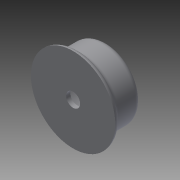
# Autodesk Inventor part: powerButtonPart2
Saved by Autodesk Inventor 2014 SP2 (Build 180246200, 246)
## iProperties
Created: 2020-04-12
Part Number: powerButtonPart2
Material: Generic
Document SubType Name: Sheet Metal
Designer: GauchoHP
Density: 1 g/cm^3
Sheet Metal Rule: Default_mm
Appearance: Default
Author: GauchoHP
Autodesk Inventor part; units mm, degrees
ref_plane "YZ Plane" through (0, 0, 0) normal (1, 0, 0) x (0, 1, 0)
ref_plane "XZ Plane" through (0, 0, 0) normal (0, 1, 0) x (-1, 0, 0)
ref_plane "XY Plane" through (0, 0, 0) normal (0, 0, 1) x (1, 0, 0)
sketch "Sketch1" plane through (0, 0, 0) normal (0, 1, 0) x (-1, 0, 0)
  circle A0 centre (0, 0) radius 9.25
  circle A1 centre (0, 0) radius 12.25
  dimension "d0" = 18.5
  dimension "d1" = 24.5
  constraints: 2 centre point, 2 coincident
  measures "d0" diameter of A0
  measures "d1" diameter of A1
extrude "Extrusion1" add sketch "Sketch1" along normal blind 10
fillet "Fillet1" radius 2 1 edges at (12.25, 10, 0)
sketch "Sketch2" plane through (0, 0, 0) normal (0, -1, 0) x (1, 0, 0)
  circle A0 centre (0, 0) radius 9.25 projected
  circle A1 centre (0, 0) radius 12.25 projected
  circle A2 centre (0, 0) radius 15
  circle A3 centre (0, 0) radius 2.5
  dimension "d6" = 30
  dimension "d9" = 5
  constraints: 2 centre point, 2 coincident
  measures "d6" diameter of A2
  measures "d9" diameter of A3
extrude "Extrusion2" add sketch "Sketch2" along normal blind 2 contours A0 | A1 | A2
fillet "Fillet3" radius 2 2 edges at (-15, 0, 0) (12.25, 0, 0)
sketch "Sketch3" plane through (0, 0, 0) normal (0, 1, 0) x (1, 0, 0)
  circle A0 centre (0, 0) radius 2.5 projected
  circle A1 centre (0, 0) radius 9.25 projected
  circle A2 centre (0, 0) radius 3.5
  dimension "d12" = 7
  constraints: 1 centre point, 1 coincident
  measures "d12" diameter of A2
extrude "Extrusion3" cut sketch "Sketch3" against normal blind 0.5 contours A2
equation "\"BendRadius\" = Thickness"
equation "\"BendReliefWidth\" = Thickness"
equation "\"BendReliefDepth\" = 0.5 * Thickness"
equation "\"CornerReliefSize\" = 4 * Thickness"
equation "\"MinimumRemnant\" = 2 * Thickness"
equation "\"TransitionRadius\" = BendRadius"
equation "\"JacobiRadiusSize\" = BendRadius"
equation "\"GapSize\" = Thickness"
equation "\"Thickness\" = 0.5"
body "Solid1"
